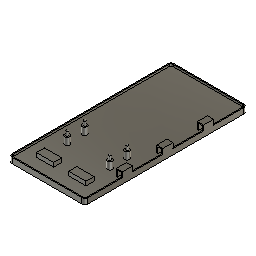
WaterSoftner v2 (Autodesk Fusion 360 design; units mm, degrees)
Autodesk Fusion 360 part; units mm, degrees
sketch "Sketch1" plane through (0, 0, 0) normal (0, 0, 1) x (1, 0, 0) in component "Component"
  line L0 (0, 0) -> (75, 0)
  line L1 (75, 0) -> (75, 160)
  line L2 (75, 160) -> (0, 160)
  line L3 (0, 160) -> (0, 0)
  dimension "d1" = 75
  dimension "d2" = 160
  constraint horizontal L0
  constraint vertical L1
  constraint horizontal L2
  constraint vertical L3
  constraint coincident L0.start L3.end
  measures "d1" distance of L0.start L0.end
  measures "d2" distance of L0.start L2.end
extrude "Extrude1" add sketch "Sketch1" along normal blind 3 in component "Component"
fillet "Fillet1" radius 3 4 edges at (75, 0, 1.5) (0, 0, 1.5) (0, 160, 1.5) (75, 160, 1.5) in component "Component"
shell "Shell1" thickness 1 removed faces 1 at (25, 105.6667, 3) in component "Component"
sketch "Sketch2" plane through (0, 0, 3) normal (0, 0, 1) x (-1, 0, 0) in component "Component"
  arc A0 (-74, -157) -> (-72, -159) centre (-72, -157) ccw
  line L0 (-74, -157) -> (-74, -3)
  arc A1 (-72, -1) -> (-74, -3) centre (-72, -3) ccw
  line L1 (-72, -1) -> (-3, -1)
  arc A2 (-1, -3) -> (-3, -1) centre (-3, -3) ccw
  line L2 (-1, -3) -> (-1, -157)
  arc A3 (-3, -159) -> (-1, -157) centre (-3, -157) ccw
  line L3 (-3, -159) -> (-72, -159)
  arc A4 (-75, -157) -> (-72, -160) centre (-72, -157) ccw
  line L4 (-72, -160) -> (-3, -160)
  arc A5 (-3, -160) -> (0, -157) centre (-3, -157) ccw
  line L5 (0, -157) -> (0, -3)
  arc A6 (0, -3) -> (-3, 0) centre (-3, -3) ccw
  line L6 (-3, 0) -> (-72, 0)
  arc A7 (-72, 0) -> (-75, -3) centre (-72, -3) ccw
  line L7 (-75, -3) -> (-75, -157)
  line L8 (-74, -157) -> (-74, -127)
  line L9 (-74, -127) -> (-75, -127)
  line L10 (-75, -127) -> (-75, -117)
  line L11 (-75, -117) -> (-74, -117)
  line L12 (-74, -117) -> (-74, -127)
  dimension "d10" = 30
  dimension "d11" = 1
  dimension "d12" = 10
  constraint coincident A0.start L0.start
  constraint parallel L0 L8
  constraint horizontal L9
  constraint vertical L10
  constraint horizontal L11
  constraint vertical L12
  measures "d10" distance of A0.start L8.end
  measures "d11" distance of L8.end L9.end
  measures "d12" distance of L8.end L11.end
extrude "Extrude3" add sketch "Sketch2" along normal blind 5 contours L0 L7 L9 L10 L11 L12 in component "Component"
sketch "Sketch3" plane through (74, 0, 0) normal (-1, 0, 0) x (0, -1, 0) in component "Component"
  line L0 (-157, 3) -> (-157, 1)
  line L1 (-157, 1) -> (-3, 1)
  line L2 (-3, 1) -> (-3, 3)
  line L3 (-3, 3) -> (-117, 3)
  line L4 (-117, 3) -> (-117, 8)
  line L5 (-117, 8) -> (-127, 8)
  line L6 (-127, 8) -> (-127, 3)
  line L7 (-127, 3) -> (-157, 3)
  line L8 (-127, 8) -> (-117, 8)
  line L9 (-117, 8) -> (-117, 7)
  line L10 (-117, 7) -> (-127, 7)
  line L11 (-127, 7) -> (-127, 8)
  constraint horizontal L8
  constraint vertical L9
  constraint horizontal L10
  constraint vertical L11
  constraint coincident L5.end L6.start
extrude "Extrude4" add sketch "Sketch3" along normal blind 5 contours L4 L5 L6 L8 L9 L10 L11 in component "Component"
sketch "Sketch4" plane through (0, 0, 8) normal (0, 0, 1) x (-1, 0, 0) in component "Component"
  line L0 (-69, -117) -> (-75, -117)
  line L1 (-75, -117) -> (-75, -127)
  line L2 (-75, -127) -> (-69, -127)
  line L3 (-69, -127) -> (-69, -117)
  line L4 (-69, -127) -> (-70, -127)
  line L5 (-70, -127) -> (-70, -117)
  line L6 (-70, -117) -> (-69, -117)
  line L7 (-69, -117) -> (-69, -127)
  dimension "d17" = 1
  constraint horizontal L4
  constraint vertical L5
  constraint horizontal L6
  constraint vertical L7
  constraint coincident L2.end L3.start
  measures "d17" distance of L2.end L4.end
extrude "Extrude5" add sketch "Sketch4" against normal up to surface (7 mm away) contours L0 L2 L3 L4 L5 L6 L7 in component "Component"
sketch "Sketch5" plane through (0, 0, 3) normal (0, 0, 1) x (-1, 0, 0) in component "Component"
  line L0 (-75, -117) -> (-74, -117)
  line L1 (-74, -117) -> (-74, -3)
  arc A0 (-72, -1) -> (-74, -3) centre (-72, -3) ccw
  line L2 (-72, -1) -> (-3, -1)
  arc A1 (-1, -3) -> (-3, -1) centre (-3, -3) ccw
  line L3 (-1, -3) -> (-1, -157)
  arc A2 (-3, -159) -> (-1, -157) centre (-3, -157) ccw
  line L4 (-3, -159) -> (-72, -159)
  arc A3 (-74, -157) -> (-72, -159) centre (-72, -157) ccw
  line L5 (-74, -157) -> (-74, -127)
  line L6 (-74, -127) -> (-75, -127)
  line L7 (-75, -127) -> (-75, -157)
  arc A4 (-75, -157) -> (-72, -160) centre (-72, -157) ccw
  line L8 (-72, -160) -> (-3, -160)
  arc A5 (-3, -160) -> (0, -157) centre (-3, -157) ccw
  line L9 (0, -157) -> (0, -3)
  arc A6 (0, -3) -> (-3, 0) centre (-3, -3) ccw
  line L10 (-3, 0) -> (-72, 0)
  arc A7 (-72, 0) -> (-75, -3) centre (-72, -3) ccw
  line L11 (-75, -3) -> (-75, -117)
  line L12 (-74, -117) -> (-74, -87)
  line L13 (-74, -87) -> (-75, -87)
  line L14 (-75, -87) -> (-75, -77)
  line L15 (-75, -77) -> (-74, -77)
  line L16 (-74, -77) -> (-74, -87)
  dimension "d20" = 30
  dimension "d21" = 1
  dimension "d22" = 10
  constraint coincident L0.end L1.start
  constraint perpendicular L0 L12
  constraint horizontal L13
  constraint vertical L14
  constraint horizontal L15
  constraint vertical L16
  measures "d20" distance of L0.end L12.end
  measures "d21" distance of L12.end L13.end
  measures "d22" distance of L12.end L15.end
extrude "Extrude6" add sketch "Sketch5" along normal blind 5 contours L1 L11 L13 L14 L15 L16 in component "Component"
sketch "Sketch6" plane through (74, 0, 0) normal (-1, 0, 0) x (0, -1, 0) in component "Component"
  line L0 (-117, 7) -> (-127, 7)
  line L1 (-127, 7) -> (-127, 3)
  line L2 (-127, 3) -> (-157, 3)
  line L3 (-157, 3) -> (-157, 1)
  line L4 (-157, 1) -> (-3, 1)
  line L5 (-3, 1) -> (-3, 3)
  line L6 (-3, 3) -> (-77, 3)
  line L7 (-77, 3) -> (-77, 8)
  line L8 (-77, 8) -> (-87, 8)
  line L9 (-87, 8) -> (-87, 3)
  line L10 (-87, 3) -> (-117, 3)
  line L11 (-117, 3) -> (-117, 7)
  line L12 (-87, 8) -> (-77, 8)
  line L13 (-77, 8) -> (-77, 7)
  line L14 (-77, 7) -> (-87, 7)
  line L15 (-87, 7) -> (-87, 8)
  dimension "d25" = 1
  constraint horizontal L12
  constraint vertical L13
  constraint horizontal L14
  constraint vertical L15
  constraint coincident L8.end L9.start
  measures "d25" distance of L8.end L14.end
extrude "Extrude7" add sketch "Sketch6" along normal blind 5 contours L7 L8 L9 L12 L13 L14 L15 in component "Component"
sketch "Sketch7" plane through (0, 0, 8) normal (0, 0, 1) x (-1, 0, 0) in component "Component"
  line L0 (-69, -77) -> (-75, -77)
  line L1 (-75, -77) -> (-75, -87)
  line L2 (-75, -87) -> (-69, -87)
  line L3 (-69, -87) -> (-69, -77)
  line L4 (-69, -87) -> (-70, -87)
  line L5 (-70, -87) -> (-70, -77)
  line L6 (-70, -77) -> (-69, -77)
  line L7 (-69, -77) -> (-69, -87)
  constraint horizontal L4
  constraint vertical L5
  constraint horizontal L6
  constraint vertical L7
  constraint coincident L0 L5.end
  constraint coincident L2.end L3.start
extrude "Extrude8" add sketch "Sketch7" against normal up to surface (7 mm away) contours L0 L2 L3 L4 L5 L6 L7 in component "Component"
sketch "Sketch8" plane through (0, 0, 3) normal (0, 0, 1) x (-1, 0, 0) in component "Component"
  line L0 (-75, -77) -> (-74, -77)
  line L1 (-74, -77) -> (-74, -3)
  arc A0 (-72, -1) -> (-74, -3) centre (-72, -3) ccw
  line L2 (-72, -1) -> (-3, -1)
  arc A1 (-1, -3) -> (-3, -1) centre (-3, -3) ccw
  line L3 (-1, -3) -> (-1, -157)
  arc A2 (-3, -159) -> (-1, -157) centre (-3, -157) ccw
  line L4 (-3, -159) -> (-72, -159)
  arc A3 (-74, -157) -> (-72, -159) centre (-72, -157) ccw
  line L5 (-74, -157) -> (-74, -127)
  line L6 (-74, -127) -> (-75, -127)
  line L7 (-75, -127) -> (-75, -157)
  arc A4 (-75, -157) -> (-72, -160) centre (-72, -157) ccw
  line L8 (-72, -160) -> (-3, -160)
  arc A5 (-3, -160) -> (0, -157) centre (-3, -157) ccw
  line L9 (0, -157) -> (0, -3)
  arc A6 (0, -3) -> (-3, 0) centre (-3, -3) ccw
  line L10 (-3, 0) -> (-72, 0)
  arc A7 (-72, 0) -> (-75, -3) centre (-72, -3) ccw
  line L11 (-75, -3) -> (-75, -77)
  line L12 (-74, -77) -> (-74, -47)
  line L13 (-74, -47) -> (-75, -47)
  line L14 (-75, -47) -> (-75, -37)
  line L15 (-75, -37) -> (-74, -37)
  line L16 (-74, -37) -> (-74, -47)
  dimension "d30" = 30
  dimension "d31" = 10
  constraint coincident L0.end L1.start
  constraint perpendicular L0 L12
  constraint horizontal L13
  constraint vertical L14
  constraint horizontal L15
  constraint vertical L16
  measures "d30" distance of L0.end L12.end
  measures "d31" distance of L12.end L15.end
extrude "Extrude9" add sketch "Sketch8" along normal blind 5 contours L1 L11 L13 L14 L15 L16 in component "Component"
sketch "Sketch9" plane through (74, 0, 0) normal (-1, 0, 0) x (0, -1, 0) in component "Component"
  line L0 (-77, 7) -> (-87, 7)
  line L1 (-87, 7) -> (-87, 3)
  line L2 (-87, 3) -> (-117, 3)
  line L3 (-117, 3) -> (-117, 7)
  line L4 (-117, 7) -> (-127, 7)
  line L5 (-127, 7) -> (-127, 3)
  line L6 (-127, 3) -> (-157, 3)
  line L7 (-157, 3) -> (-157, 1)
  line L8 (-157, 1) -> (-3, 1)
  line L9 (-3, 1) -> (-3, 3)
  line L10 (-3, 3) -> (-37, 3)
  line L11 (-37, 3) -> (-37, 8)
  line L12 (-37, 8) -> (-47, 8)
  line L13 (-47, 8) -> (-47, 3)
  line L14 (-47, 3) -> (-77, 3)
  line L15 (-77, 3) -> (-77, 7)
  line L16 (-47, 8) -> (-37, 8)
  line L17 (-37, 8) -> (-37, 7)
  line L18 (-37, 7) -> (-47, 7)
  line L19 (-47, 7) -> (-47, 8)
  dimension "d34" = 1
  constraint horizontal L16
  constraint vertical L17
  constraint horizontal L18
  constraint vertical L19
  constraint coincident L12.end L13.start
  measures "d34" distance of L12.end L18.end
extrude "Extrude10" add sketch "Sketch9" along normal blind 5 contours L11 L12 L13 L16 L17 L18 L19 in component "Component"
sketch "Sketch10" plane through (0, 0, 8) normal (0, 0, 1) x (-1, 0, 0) in component "Component"
  line L0 (-69, -37) -> (-75, -37)
  line L1 (-75, -37) -> (-75, -47)
  line L2 (-75, -47) -> (-69, -47)
  line L3 (-69, -47) -> (-69, -37)
  line L4 (-69, -47) -> (-70, -47)
  line L5 (-70, -47) -> (-70, -37)
  line L6 (-70, -37) -> (-69, -37)
  line L7 (-69, -37) -> (-69, -47)
  constraint horizontal L4
  constraint vertical L5
  constraint horizontal L6
  constraint vertical L7
  constraint coincident L0 L5.end
  constraint coincident L2.end L3.start
extrude "Extrude11" add sketch "Sketch10" against normal up to surface (7 mm away) contours L0 L2 L3 L4 L5 L6 L7 in component "Component"
sketch "Sketch11" plane through (0, 0, 1) normal (0, 0, 1) x (-1, 0, 0) in component "Component"
  line L0 (-70, -37) -> (-69, -37)
  line L1 (-69, -37) -> (-69, -47)
  line L2 (-69, -47) -> (-70, -47)
  line L3 (-70, -47) -> (-70, -37)
  line L4 (-70, -77) -> (-69, -77)
  line L5 (-69, -77) -> (-69, -87)
  line L6 (-69, -87) -> (-70, -87)
  line L7 (-70, -87) -> (-70, -77)
  line L8 (-70, -117) -> (-69, -117)
  line L9 (-69, -117) -> (-69, -127)
  line L10 (-69, -127) -> (-70, -127)
  line L11 (-70, -127) -> (-70, -117)
  arc A0 (-74, -157) -> (-72, -159) centre (-72, -157) ccw
  line L12 (-72, -159) -> (-3, -159)
  arc A1 (-3, -159) -> (-1, -157) centre (-3, -157) ccw
  line L13 (-1, -157) -> (-1, -3)
  arc A2 (-1, -3) -> (-3, -1) centre (-3, -3) ccw
  line L14 (-3, -1) -> (-72, -1)
  arc A3 (-72, -1) -> (-74, -3) centre (-72, -3) ccw
  line L15 (-74, -3) -> (-74, -157)
  line L16 (-72, -1) -> (-72, -14)
  line L17 (-3, -1) -> (-3, -14)
  line L18 (-3, -14) -> (-72, -14)
  line L19 (-72, -14) -> (-72, -22)
  line L20 (-72, -22) -> (-3, -22)
  line L21 (-3, -22) -> (-3, -14)
  dimension "d39" = 13
  dimension "d40" = 13
  dimension "d41" = 8
  constraint vertical L16
  constraint coincident L14.end A3.start
  constraint vertical L17
  constraint coincident A2.end L14.start
  constraint horizontal L18
  constraint vertical L19
  constraint horizontal L20
  constraint vertical L21
  measures "d39" distance of L14.end L16.end
  measures "d40" distance of A2.end L17.end
  measures "d41" distance of L17.end L20.end
extrude "Extrude12" add sketch "Sketch11" along normal blind 3 contours L18 L19 L20 L21 in component "Component"
extrude "Extrude13" cut 1 faces at (72, 16.6667, 2) along direction (-1, 0, 0) blind 10 in component "Component"
extrude "Extrude14" cut 1 faces at (3, 19.3333, 2) along direction (1, 0, 0) blind 10 in component "Component"
sketch "Sketch12" plane through (0, 0, 1) normal (0, 0, 1) x (-1, 0, 0) in component "Component"
  line L0 (-13, -22) -> (-62, -22)
  line L1 (-62, -22) -> (-62, -14)
  line L2 (-62, -14) -> (-13, -14)
  line L3 (-13, -14) -> (-13, -22)
  line L4 (-70, -37) -> (-69, -37)
  line L5 (-69, -37) -> (-69, -47)
  line L6 (-69, -47) -> (-70, -47)
  line L7 (-70, -47) -> (-70, -37)
  line L8 (-70, -77) -> (-69, -77)
  line L9 (-69, -77) -> (-69, -87)
  line L10 (-69, -87) -> (-70, -87)
  line L11 (-70, -87) -> (-70, -77)
  line L12 (-70, -117) -> (-69, -117)
  line L13 (-69, -117) -> (-69, -127)
  line L14 (-69, -127) -> (-70, -127)
  line L15 (-70, -127) -> (-70, -117)
  arc A0 (-74, -157) -> (-72, -159) centre (-72, -157) ccw
  line L16 (-72, -159) -> (-3, -159)
  arc A1 (-3, -159) -> (-1, -157) centre (-3, -157) ccw
  line L17 (-1, -157) -> (-1, -3)
  arc A2 (-1, -3) -> (-3, -1) centre (-3, -3) ccw
  line L18 (-3, -1) -> (-72, -1)
  arc A3 (-72, -1) -> (-74, -3) centre (-72, -3) ccw
  line L19 (-74, -3) -> (-74, -157)
  line L20 (-37.5, -1) -> (-37.5, -41) construction
  line L21 (-37.5, -41) -> (-58.5, -41) construction
  line L22 (-37.5, -41) -> (-16.5, -41) construction
  line L23 (-16.5, -41) -> (-58.5, -41) construction
  line L24 (-58.5, -41) -> (-58.5, -58.2) construction
  line L25 (-58.5, -58.2) -> (-16.5, -58.2) construction
  line L26 (-16.5, -58.2) -> (-16.5, -41) construction
  circle A4 centre (-16.5, -58.2) radius 2.5
  circle A5 centre (-58.5, -58.2) radius 2.5
  circle A6 centre (-16.5, -41) radius 2.5
  circle A7 centre (-58.5, -41) radius 2.5
  dimension "d48" = 40
  dimension "d49" = 21
  dimension "d50" = 21
  dimension "d51" = 42
  dimension "d52" = 17.2
  dimension "d53" = 5
  dimension "d54" = 5
  dimension "d55" = 5
  dimension "d56" = 5
  constraint midpoint L18 L20.start
  constraint perpendicular L0 L20
  constraint perpendicular L20 L21
  constraint perpendicular L20 L22
  constraint horizontal L23
  constraint vertical L24
  constraint horizontal L25
  constraint vertical L26
  constraint coincident L25.end L26.start
  constraint coincident L24.end L25.start
  constraint coincident L22.end L23.start
  constraint coincident L21.end L23.end
  measures "d48" distance of L20.start L20.end
  measures "d49" distance of L20.end L21.end
  measures "d50" distance of L20.end L22.end
  measures "d51" distance of L22.end L21.end
  measures "d52" distance of L22.end L25.end
  measures "d53" diameter of A4
  measures "d54" diameter of A5
  measures "d55" diameter of A6
  measures "d56" diameter of A7
extrude "Extrude15" add sketch "Sketch12" along normal blind 7 contours A4 | A5 | A6 | A7 in component "Component"
sketch "Sketch13" plane through (0, 0, 8) normal (0, 0, 1) x (-1, 0, 0) in component "Component"
  circle A0 centre (-16.5, -58.2) radius 2.5
  circle A1 centre (-16.5, -58.2) radius 1.1
  circle A2 centre (-58.5, -58.2) radius 1.1
  circle A3 centre (-58.5, -58.2) radius 2.5
  circle A4 centre (-16.5, -41) radius 1.1
  circle A5 centre (-16.5, -41) radius 2.5
  circle A6 centre (-58.5, -41) radius 1.1
  circle A7 centre (-58.5, -41) radius 2.5
  dimension "d59" = 2.2
  dimension "d60" = 2.2
  dimension "d61" = 2.2
  dimension "d62" = 2.2
  constraint concentric A0 A1
  constraint concentric A2 A3
  constraint concentric A4 A5
  constraint concentric A6 A7
  measures "d59" diameter of A1
  measures "d60" diameter of A2
  measures "d61" diameter of A4
  measures "d62" diameter of A6
extrude "Extrude16" add sketch "Sketch13" along normal blind 5 contours A1 | A2 | A4 | A6 in component "Component"
fillet "Fillet2" radius 1 4 edges at (59.5256, 41.3978, 13) (59.5256, 58.5978, 13) (17.5256, 58.5978, 13) (17.5256, 41.3978, 13) in component "Component"
sketch "Sketch14" plane through (0, 0, 4) normal (0, 0, 1) x (-1, 0, 0) in component "Component"
  line L0 (-13, -22) -> (-13, -14)
  line L1 (-13, -14) -> (-62, -14)
  line L2 (-62, -14) -> (-62, -22)
  line L3 (-62, -22) -> (-13, -22)
  line L4 (-37.5, -22) -> (-37.5, -14) construction
  line L5 (-45, -14) -> (-30, -14)
  line L6 (-30, -14) -> (-30, -22)
  line L7 (-30, -22) -> (-45, -22)
  line L8 (-45, -22) -> (-45, -14)
  line L9 (-45, -14) -> (-30, -22) construction
  line L10 (-30, -14) -> (-45, -22) construction
  point P0 (-37.5, -18)
  dimension "d67" = 15
  constraint midpoint L3 L4.start
  constraint midpoint L1 L4.end
  constraint horizontal L5
  constraint perpendicular L5 L6
  constraint parallel L5 L7
  constraint parallel L6 L8
  constraint coincident L9 P0
  constraint coincident L10 P0
  constraint midpoint L4 P0
  measures "d67" distance of L6.end L7.end
extrude "Extrude17" cut sketch "Sketch14" against normal up to surface (3 mm away) contours L1 L3 L5 L6 L7 L8 in component "Component"
extrude "Extrude18" add 1 faces at (25, 105.6667, 0) along direction (0, 0, -1) blind 2.5 in component "Component"
extrude "Extrude19" add 2 faces at (24.3333, 16.6667, 4) (56.3333, 19.3333, 4) along direction (0, 0, 1) blind 1 in component "Component"
component "Component" placed x (1, 0, 0) y (0, 1, 0) z (0, 0, 1) at (0, 0, 0)
